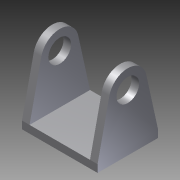
# Autodesk Inventor part: manipulator pnumaitic pivot
Saved by Autodesk Inventor 2012 (Build 160160000, 160)
## iProperties
Created: 2013-09-04
Part Number: manipulator pnumaitic pivot
Material: Default
Document SubType Name: Modeling
Designer: Bryce
Density: 1 g/cm^3
Author: Bryce
Autodesk Inventor part; units mm, degrees
ref_plane "YZ Plane" through (0, 0, 0) normal (1, 0, 0) x (0, 1, 0)
ref_plane "XZ Plane" through (0, 0, 0) normal (0, 1, 0) x (-1, 0, 0)
ref_plane "XY Plane" through (0, 0, 0) normal (0, 0, 1) x (1, 0, 0)
sketch "Sketch1" plane through (0, 0, 0) normal (0, 0, 1) x (1, 0, 0)
  line L0 (0, 0) -> (31.75, 0)
  line L1 (31.75, 0) -> (31.75, 31.75)
  line L2 (0, 31.75) -> (0, 0)
  line L3 (28.575, 31.75) -> (28.575, 3.175)
  line L4 (28.575, 3.175) -> (3.175, 3.175)
  line L5 (3.175, 3.175) -> (3.175, 31.75)
  line L6 (31.75, 31.75) -> (28.575, 31.75)
  line L7 (3.175, 31.75) -> (0, 31.75)
  dimension "d0" = 31.75
  dimension "d1" = 31.75
  dimension "d2" = 3.175
  dimension "d3" = 3.175
  dimension "d4" = 3.175
  constraints: 16 end point, 4 parallel, 1 collinear, 1 horizontal, 1 perpendicular
  measures "d0" distance of L2.start L0.start
  measures "d1" distance of L0.start L0.end
  measures "d2" distance between parallel lines of L2 L5
  measures "d3" distance between parallel lines of L4 L0
  measures "d4" distance between parallel lines of L1 L3
extrude "Extrusion1" add sketch "Sketch1" along normal blind 25.4
sketch "Sketch2" plane through (31.75, 0, 0) normal (1, 0, 0) x (0, 0, -1)
  line L0 (-25.4, 31.75) -> (-25.4, 0) projected
  line L1 (0, 0) -> (-25.4, 0) projected
  line L2 (0, 0) -> (0, 31.75) projected
  line L3 (0, 31.75) -> (-25.4, 31.75) projected
  arc A0 (-4.9503, 25.5287) -> (-20.4497, 25.5287) centre (-12.7, 23.8125) ccw
  line L4 (-25.4, 3.175) -> (-20.4497, 25.5287)
  line L5 (0, 3.175) -> (-4.9503, 25.5287)
  circle A1 centre (-12.7, 23.8125) radius 4.7625
  dimension "d7" = 15.875
  dimension "d8" = 3.175
  dimension "d9" = 9.525
  dimension "d10" = 12.7
  constraints: 4 end point, 3 tangent, 2 centre point, 2 point on circle, 2 point on line, 1 coincident, 1 horizontal alignment
  measures "d7" diameter of A0
  measures "d8" distance of L0.end L4.start
  measures "d9" diameter of A1
  measures "d10" distance from line of A0.centre L0
extrude "Extrusion2" cut sketch "Sketch2" against normal through all contours L3 A0 L4 L0 | L3 L2 L5 A0 | A1
equation "\"d3\" = d2"
equation "\"d4\" = d3"
body "Solid1"
